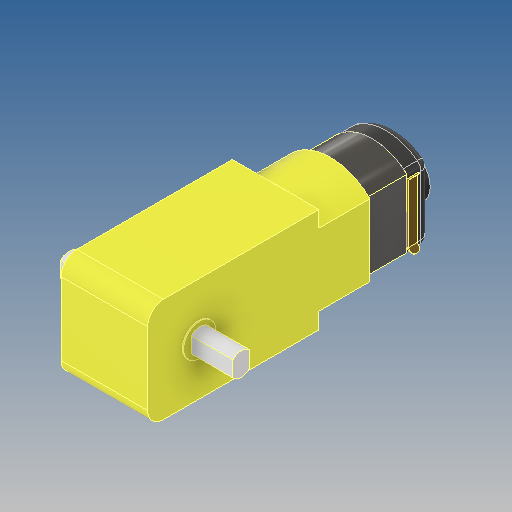
# Autodesk Inventor part: Arduino Gear Motor
Saved by Autodesk Inventor 2020 (Build 240168000, 168)
## iProperties
Created: 2018-07-22
Part Number: Arduino Gear Motor
Material: PBT Plastic
Document SubType Name: Modeling
Designer: admin1
Density: 1.31 g/cm^3
Appearance: Smooth - Yellow
Author: admin1
Autodesk Inventor part; units mm, degrees
ref_plane "YZ Plane" through (0, 0, 0) normal (1, 0, 0) x (0, 1, 0)
ref_plane "XZ Plane" through (0, 0, 0) normal (0, 1, 0) x (-1, 0, 0)
ref_plane "XY Plane" through (0, 0, 0) normal (0, 0, 1) x (1, 0, 0)
sketch "Sketch1" plane through (0, 0, 0) normal (0, 0, 1) x (1, 0, 0)
  line L0 (9.35, -11.25) -> (-9.35, -11.25)
  line L1 (-9.35, -11.25) -> (-9.35, 11.25)
  line L2 (-9.35, 11.25) -> (9.35, 11.25)
  line L3 (9.35, 11.25) -> (9.35, -11.25)
  line L4 (9.35, -11.25) -> (-9.35, 11.25) construction
  line L5 (-9.35, -11.25) -> (9.35, 11.25) construction
  point P0 (0, 0)
  dimension "d0" = 18.7
  dimension "d1" = 22.5
  constraints: 12 end point, 2 midpoint, 2 parallel, 1 horizontal, 1 perpendicular
  measures "d0" distance of L1.end L2.end
  measures "d1" distance of L2.end L0.start
extrude "Extrusion1" add sketch "Sketch1" against normal blind 37
fillet "Fillet1" radius 3.4 2 edges at (0, 11.25, 0) (0, -11.25, 0)
sketch "Sketch2" plane through (0, 0, -37) normal (0, 0, -1) x (-1, 0, 0)
  line L0 (-9.35, 11.25) -> (-9.35, -11.25) projected
  line L1 (9.35, 11.25) -> (-9.35, 11.25) projected
  line L2 (-9.35, -11.25) -> (9.35, -11.25) projected
  arc A0 (7.65, 7.75) -> (-9.35, 7.75) centre (-0.85, -0.8214) ccw
  arc A1 (-9.35, -7.75) -> (7.65, -7.75) centre (-0.85, 0.8214) ccw
  line L3 (7.65, -7.75) -> (7.65, 7.75)
  point P0 (0, 0)
  dimension "d5" = 3.5
  dimension "d6" = 3.5
  dimension "d7" = 17
  constraints: 4 point on circle, 2 centre point, 2 end point, 2 horizontal alignment, 2 point on line, 2 tangent, 1 vertical
  measures "d5" distance from line of A1.start L2
  measures "d6" distance from line of L1 A0.end
  measures "d7" distance between parallel lines of L0 L3
extrude "Extrusion2" add sketch "Sketch2" along normal blind 11 contours A0 L3 A1 L0
sketch "Sketch3" plane through (0, 0, -48) normal (0, 0, -1) x (-1, 0, 0)
  arc A0 (7.65, 7.75) -> (-9.35, 7.75) centre (-0.85, -0.8214) ccw projected
  line L0 (-9.35, 7.75) -> (-9.35, -7.75) projected
  arc A1 (-9.35, -7.75) -> (7.65, -7.75) centre (-0.85, 0.8214) ccw projected
  line L1 (7.65, -7.75) -> (7.65, 7.75) projected
  arc A2 (6.65, 7.3227) -> (-8.35, 7.3227) centre (-0.85, -0.8214) ccw
  line L2 (6.65, 7.3227) -> (6.65, -7.3227)
  arc A3 (-8.35, -7.3227) -> (6.65, -7.3227) centre (-0.85, 0.8214) ccw
  line L3 (-8.35, -7.3227) -> (-8.35, 7.3227)
  point P0 (0, 0)
  dimension "d10" = 1
  constraints: 4 end point, 4 point on circle, 2 centre point, 3 other
  measures "d10" radial gap between concentric circles of A0 A2
extrude "Extrusion3" add sketch "Sketch3" along normal blind 9 contours L2 A3 L3 A2
sketch "Sketch4" plane through (0, 0, -57) normal (0, 0, -1) x (-1, 0, 0)
  arc A0 (6.65, 7.3227) -> (-8.35, 7.3227) centre (-0.85, -0.8214) ccw projected
  line L0 (-8.35, 7.3227) -> (-8.35, -7.3227) projected
  arc A1 (-8.35, -7.3227) -> (6.65, -7.3227) centre (-0.85, 0.8214) ccw projected
  line L1 (6.65, -7.3227) -> (6.65, 7.3227) projected
  point P0 (0, 0)
extrude "Extrusion4" add sketch "Sketch4" along normal blind 5 separate body
sketch "Sketch5" plane through (9.35, -7.85, 0) normal (1, 0, 0) x (0, 0, -1)
  circle A0 centre (11, 7.85) radius 3.5
  line L0 (0, 15.7) -> (0, 0) projected
  point P0 (0, 7.85)
  point P1 (0, 7.85)
  dimension "d15" = 11
  dimension "d16" = 7
  constraints: 1 centre point, 1 horizontal alignment, 1 midpoint
  measures "d15" distance from line of L0 A0.centre
  measures "d16" diameter of A0
extrude "Extrusion5" add sketch "Sketch5" along normal blind 0.25 bodies 1
sketch "Sketch6" plane through (9.6, 0, -11) normal (1, 0, 0) x (0, 0, -1)
  circle A0 centre (0, 0) radius 3.5 projected
  circle A1 centre (0, 0) radius 2.5
  point P0 (-11, 0)
  dimension "d19" = 5
  constraints: 1 centre point
  measures "d19" diameter of A1
extrude "Extrusion6" add sketch "Sketch6" along normal blind 9 contours A1 bodies 1
sketch "Sketch7" plane through (18.6, 0, -11) normal (1, 0, 0) x (0, 0, -1)
  circle A0 centre (0, 0) radius 2.5 projected
  circle A1 centre (0, 0) radius 2.5 projected
  line L0 (1.85, 1.6815) -> (1.85, -1.6815)
  line L1 (-1.85, -1.6815) -> (-1.85, 1.6815)
  line L2 (0, 0) -> (0, 2.5) construction
  point P0 (-11, 0)
  dimension "d22" = 3.7
  dimension "d23" = 1.85
  dimension "angle" = 0
  constraints: 6 end point, 5 point on circle, 1 parallel, 1 vertical
  measures "d22" distance between parallel lines of L1 L0
  measures "d23" distance from line of L0 A0.centre
  measures "angle" angle of L1 L2
extrude "Extrusion7" cut sketch "Sketch7" against normal blind 9 contours A0 L0 | L1 A0 bodies 1
mirror "Mirror1" about plane through (0, 0, 0) normal (1, 0, 0) of "Extrusion6", "Extrusion5", "Extrusion7" bodies 1
sketch "Sketch8" plane through (-9.35, -11.25, -37) normal (-1, 0, 0) x (0, 0, 1)
  circle A0 centre (15, 11.25) radius 2
  line L0 (37, 3.4) -> (37, 19.1) projected
  point P0 (37, 11.25)
  point P1 (37, 11.25)
  dimension "d27" = 4
  dimension "d28" = 22
  constraints: 1 centre point, 1 horizontal alignment, 1 midpoint
  measures "d27" diameter of A0
  measures "d28" distance from line of L0 A0.centre
extrude "Extrusion8" add sketch "Sketch8" along normal blind 1.5 bodies 1
fillet "Fillet2" radius 2 8 edges at (8.35, 0, -62) (0.85, 10.25, -62) (-6.65, 0, -62) (0.85, -10.25, -62) (8.35, 7.3227, -59.5) (8.35, -7.3227, -59.5) (-6.65, 7.3227, -59.5) (-6.65, -7.3227, -59.5)
sketch "Sketch9" plane through (0, 0, -62) normal (0, 0, -1) x (-1, 0, 0)
  arc A0 (-6.35, -6.3925) -> (4.65, -6.3925) centre (-0.85, 0.8214) ccw projected
  line L0 (4.65, 6.3925) -> (4.65, -6.3925) projected
  arc A1 (4.65, 6.3925) -> (-6.35, 6.3925) centre (-0.85, -0.8214) ccw projected
  line L1 (-6.35, -6.3925) -> (-6.35, 6.3925) projected
  circle A2 centre (-0.85, 0) radius 5
  line L2 (3.4, 2.6339) -> (3.4, -2.6339)
  point P0 (0, 0)
  dimension "d32" = 10
  dimension "d33" = 4.25
  constraints: 2 end point, 2 point on circle, 1 centre point, 1 horizontal alignment, 1 vertical, 1 vertical alignment
  measures "d32" diameter of A2
  measures "d33" distance from line of A2.centre L2
extrude "Extrusion9" add sketch "Sketch9" along normal blind 2.5 contours L2 A2 picked at (0.3293, -0.2048) bodies 2
sketch "Sketch10" plane through (0, 0, -64.5) normal (0, 0, -1) x (-1, 0, 0)
  arc A0 (3.4, 2.6339) -> (3.4, -2.6339) centre (-0.85, 0) ccw projected
  circle A1 centre (-0.85, 0) radius 1
  point P0 (0, 0)
  dimension "d36" = 2
  constraints: 1 centre point, 1 coincident
  measures "d36" diameter of A1
extrude "Extrusion10" add sketch "Sketch10" along normal blind 1 separate body
sketch "Sketch11" plane through (0, 0, -64.5) normal (0, 0, -1) x (-1, 0, 0)
  line L0 (-8.35, 6.3925) -> (-8.35, -6.3925) projected
  line L1 (-8.35, -7.3227) -> (-8.35, 7.3227) projected
  line L2 (-8.35, 6.3925) -> (-9.35, 7.5)
  line L3 (-9.35, 7.5) -> (-9.5356, 7.3325)
  line L4 (-9.5356, 7.3325) -> (-8.6, 6.2963)
  line L5 (-8.6, 6.2963) -> (-8.6, -6.2963)
  line L6 (-8.6, -6.2963) -> (-9.5356, -7.3325)
  line L7 (-9.5356, -7.3325) -> (-9.35, -7.5)
  line L8 (-9.35, -7.5) -> (-8.35, -6.3925)
  point P0 (0, 0)
  point P1 (-8.6, 0)
  dimension "d39" = 0.25
  dimension "d40" = 15
  dimension "d41" = 0.25
  dimension "d42" = 1
  constraints: 14 end point, 4 perpendicular, 2 vertical alignment, 1 equal length, 1 horizontal alignment, 1 midpoint, 1 point on line, 1 vertical
  measures "d39" distance of L2.end L3.end
  measures "d40" distance of L7.end L2.end
  measures "d41" distance between parallel lines of L0 L5
  measures "d42" distance from line of L0 L2.end
extrude "Extrusion11" add sketch "Sketch11" along normal blind 2 from surface at -7.5 separate body
fillet "Fillet3" radius 1 4 edges at (9.4428, 7.4162, -59) (9.4428, 7.4162, -57) (9.4428, -7.4162, -59) (9.4428, -7.4162, -57)
equation "\"d5\" = d6"
equation "\"d23\" = 0.5 * d22"
equation "\"d41\" = d39"
body "Solid1"
body "Solid2"
body "Solid3"
body "Solid4"
